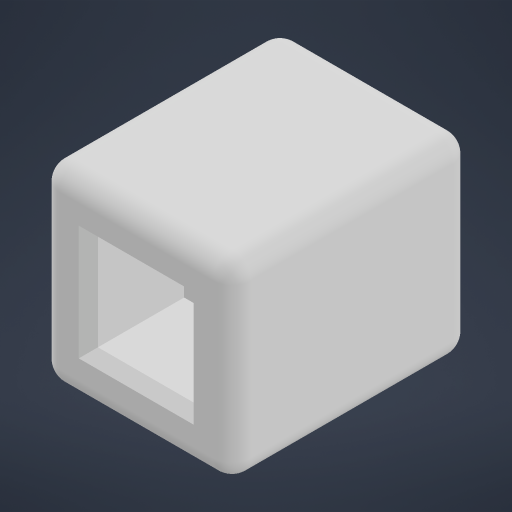
# Autodesk Inventor part: Hole_TestFits
Saved by Autodesk Inventor 2024 (Build 280153000, 153)
## iProperties
Created: 2023-07-01
Part Number: Hole_TestFits
Material: Generic
Document SubType Name: Modeling
Designer: User
Density: 1 g/cm^3
Appearance: Default
Author: User
Autodesk Inventor part; units mm, degrees
ref_plane "YZ Plane" through (0, 0, 0) normal (1, 0, 0) x (0, 1, 0)
ref_plane "XZ Plane" through (0, 0, 0) normal (0, 1, 0) x (-1, 0, 0)
ref_plane "XY Plane" through (0, 0, 0) normal (0, 0, 1) x (1, 0, 0)
sketch "Sketch14" plane through (0, 0, 0) normal (0, 0, 1) x (1, 0, 0)
  line L0 (0, 0) -> (-20, 0)
  line L1 (-20, 0) -> (-20, 20)
  line L2 (-20, 20) -> (0, 20)
  line L3 (0, 20) -> (0, 0)
  line L4 (-5, 5) -> (-10, 5)
  line L5 (-10, 5) -> (-10, 10)
  line L6 (-10, 10) -> (-5, 10)
  line L7 (-5, 10) -> (-5, 5)
  dimension "d71" = 20
  dimension "d72" = 20
  dimension "d73" = 5
  dimension "d74" = 5
  constraints: 16 end point, 4 parallel, 2 horizontal, 2 perpendicular
  measures "d71" distance of L1.end L2.end
  measures "d72" distance of L0.end L1.end
  measures "d73" distance of L5.end L6.end
  measures "d74" distance of L4.end L5.end
extrude "Extrusion9" add sketch "Sketch14" along normal blind 25 contours L0 L1 L2 L3 | L4 L5 L6 L7
fillet "Fillet1" radius 2 12 edges at (-20, 20, 12.5) (-20, 10, 0) (-20, 0, 12.5) (-20, 10, 25) (0, 10, 25) (-10, 20, 25) (0, 20, 12.5) (-10, 20, 0) (-10, 0, 25) (0, 10, 0) (0, 0, 12.5) (-10, 0, 0)
sketch "Sketch24" plane through (0, 0, 25) normal (0, 0, 1) x (1, 0, 0)
  line L0 (-15, 15) -> (-5, 15)
  line L1 (-5, 15) -> (-5, 5)
  line L2 (-5, 5) -> (-15, 5)
  line L3 (-15, 5) -> (-15, 15)
  point P0 (0, 0)
  dimension "d176" = 10
  dimension "d177" = 10
  constraints: 8 end point, 2 parallel, 1 horizontal, 1 perpendicular
  measures "d176" distance of L1.end L2.end
  measures "d177" distance of L0.end L1.end
extrude "Extrusion16" cut sketch "Sketch24" against normal blind 10
sketch "Sketch31" plane through (0, 0, 0) normal (0, 0, -1) x (-1, 0, 0)
  line L0 (5, 5) -> (15, 5)
  line L1 (15, 5) -> (15, 15)
  line L2 (15, 15) -> (5, 15)
  line L3 (5, 15) -> (5, 5)
  point P0 (0, 0)
  dimension "d231" = 10
  dimension "d232" = 10
  constraints: 8 end point, 2 parallel, 1 horizontal, 1 perpendicular
  measures "d231" distance of L2.end L1.end
  measures "d232" distance of L1.end L0.end
extrude "Extrusion18" cut sketch "Sketch31" against normal blind 10
chamfer "Chamfer15" distance 1 angle 45 8 edges at (-10, 15, 0) (-15, 10, 0) (-10, 5, 0) (-5, 10, 0) (-10, 15, 25) (-5, 10, 25) (-10, 5, 25) (-15, 10, 25)
body "Solid4"
